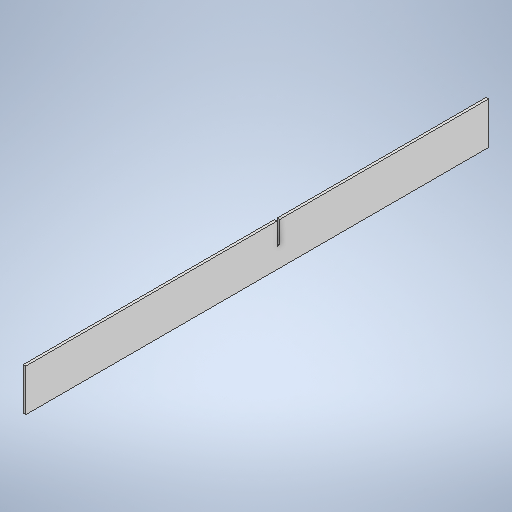
# Autodesk Inventor part: BSH 042 stringer floor
Saved by Autodesk Inventor 2025 (Build 290162010, 162A)
## iProperties
Created: 2024-07-23
Part Number: BSH 042 stringer floor
Material: Stainless Steel
Document SubType Name: Sheet Metal
Designer: pokla
Density: 8 g/cm^3
Sheet Metal Rule: AISI304 3mm Die 32
Appearance: Default
Mass: 658.243 g
Surface Area: 586.108 cm^2
Volume: 82.2804 cm^3
Author: pokla
Autodesk Inventor part; units mm, degrees
ref_plane "YZ Plane" through (0, 0, 0) normal (1, 0, 0) x (0, 1, 0)
ref_plane "XZ Plane" through (0, 0, 0) normal (0, 1, 0) x (-1, 0, 0)
ref_plane "XY Plane" through (0, 0, 0) normal (0, 0, 1) x (1, 0, 0)
sketch "Sketch1" plane through (0, 0, 0) normal (1, 0, 0) x (0, 1, 0)
  line L0 (-275.1, 50) -> (275.1, 50)
  line L1 (275.1, 50) -> (275.1, 0)
  line L2 (275.1, 0) -> (-275.1, 0)
  line L3 (-275.1, 0) -> (-275.1, 50)
  point P0 (0, 0)
  point P1 (0, 0)
  dimension "d0" = 50
  dimension "d1" = 550.2
  measures "d0" distance of L2.end L0.start
  measures "d1" distance of L0.start L0.end
extrude "Plate1" add sketch "Sketch1" against normal blind 3
sketch "Sketch2" plane through (0, 0, 0) normal (1, 0, 0) x (0, 0, -1)
  line L0 (-50, 275.1) -> (-50, -275.1) projected
  line L1 (-50, 23.5) -> (-24, 23.5)
  line L2 (-24, 23.5) -> (-24, 26.7)
  line L3 (-24, 26.7) -> (-50, 26.7)
  line L4 (-50, 26.7) -> (-50, 23.5)
  point P0 (0, 0)
  point P1 (-50, 26.7)
  point P2 (-50, 25.1)
  dimension "d4" = 3.2
  dimension "d5" = 26
  dimension "d14" = 298.6
  constraints: 8 end point, 2 parallel, 1 horizontal, 1 midpoint, 1 perpendicular, 1 point on line
  measures "d4" distance of L1.end L2.end
  measures "d5" distance of L1.start L1.end
  measures "d14" distance of L0.end L1.start
extrude "Extrusion1" cut sketch "Sketch2" against normal through all
equation "\"d2\" = Thickness"
equation "\"BendReliefWidth\" = Thickness"
equation "\"BendReliefDepth\" = 0.5 * Thickness"
equation "\"CornerReliefSize\" = 4 * Thickness"
equation "\"MinimumRemnant\" = 2 * Thickness"
equation "\"TransitionRadius\" = BendRadius"
equation "\"JacobiRadiusSize\" = BendRadius"
equation "\"GapSize\" = Thickness"
equation "\"Thickness\" = 3"
equation "\"BendRadius\" = 5"
body "Solid1"
